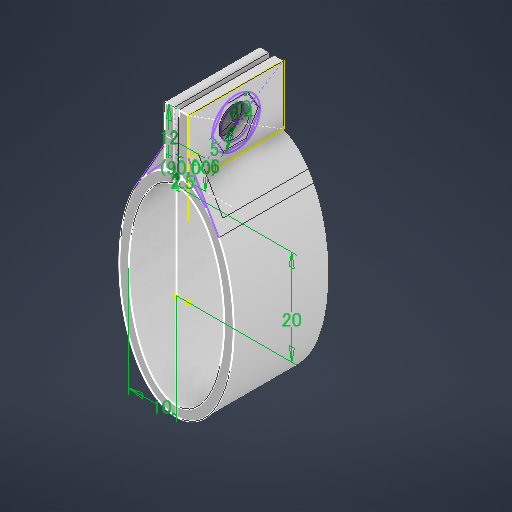
# Autodesk Inventor part: default
Saved by Autodesk Inventor 2025.2 (Build 292293000, 293)
## iProperties
Created: 2024-07-26
Part Number: default
Material: 一般
Document SubType Name: Modeling
Designer: ktamu
Density: 1 g/cm^3
Appearance: 既定
Author: ktamu
Autodesk Inventor part; units mm, degrees
note: some values were not read from the file. Chosen so that the rebuilt part matches the saved one: offset side.
ref_plane "YZ Plane" through (0, 0, 0) normal (1, 0, 0) x (0, 1, 0)
ref_plane "XZ Plane" through (0, 0, 0) normal (0, 1, 0) x (-1, 0, 0)
ref_plane "XY Plane" through (0, 0, 0) normal (0, 0, 1) x (1, 0, 0)
sketch "スケッチ1" plane through (0, 0, 0) normal (0, 0, 1) x (1, 0, 0)
  ellipse E0 centre (0, 0) end of major axis (0, -20) minor radius 10
  line L0 (0, 0) -> (0, 22)
  line L1 (0, 0) -> (0, -22)
  line L2 (0, 22) -> (0, 34)
  line L3 (0, 22) -> (12, 22) construction
  line L4 (0, 34) -> (2.5, 34)
  line L5 (2.5, 34) -> (2.5, 22)
  line L6 (2.5, 22) -> (0, 22)
  line L7 (0, 22) -> (0, 34)
  line L8 (0, 34) -> (-2.5, 34)
  line L9 (-2.5, 34) -> (-2.5, 22)
  line L10 (-2.5, 22) -> (0, 22)
  line L11 (-0.5, 34) -> (0.5, 34)
  line L12 (0.5, 34) -> (0.5, 22)
  line L13 (0.5, 22) -> (-0.5, 22)
  line L14 (-0.5, 22) -> (-0.5, 34)
  line L15 (-0.5, 34) -> (0.5, 22) construction
  line L16 (0.5, 34) -> (-0.5, 22) construction
  line L17 (2.5, 26.1957) -> (8.883, 14.9903)
  line L18 (-2.5, 26.1957) -> (-8.883, 14.9903)
  line L19 (-0.5, 22) -> (-0.5, 19.975)
  line L20 (0.5, 22) -> (0.5, 19.975)
  line L21 (-6.1194, 19.0632) -> (-2.5, 23.108)
  line L22 (6.1194, 19.0632) -> (2.5, 23.108)
  line L23 (-2.5, 22) -> (-2.5, 21.4925)
  line L24 (2.5, 22) -> (2.5, 21.3781)
  spline S0 degree 5 poles (0, -22) (1.1169, -22.0001) (2.2373, -21.7769) (3.2884, -21.3301) (5.3155, -20.0562) (6.9198, -18.2708) (7.6546, -17.2439) (9.0536, -14.8879) (10.0679, -12.3406) (10.5239, -10.9338) (11.3093, -7.9323) (11.7649, -4.8627) (11.9216, -3.2452) (12.0784, 0) (11.9216, 3.2451) (11.765, 4.8626) (11.3092, 7.9322) (10.524, 10.9338) (10.0678, 12.3407) (9.0538, 14.888) (7.6543, 17.244) (6.9201, 18.2709) (5.3148, 20.0562) (3.2891, 21.3301) (2.2357, 21.777) (0, 22.223) (-2.2357, 21.777) (-3.2891, 21.3301) (-5.3148, 20.0562) (-6.9201, 18.2709) (-7.6543, 17.244) (-9.0538, 14.888) (-10.0678, 12.3407) (-10.524, 10.9338) (-11.3092, 7.9322) (-11.765, 4.8626) (-11.9216, 3.2451) (-12.0784, 0) (-11.9216, -3.2452) (-11.7649, -4.8627) (-11.3093, -7.9323) (-10.5239, -10.9338) (-10.0679, -12.3406) (-9.0536, -14.8879) (-7.6546, -17.2439) (-6.9198, -18.2708) (-5.3155, -20.0562) (-3.2884, -21.3301) (-2.2373, -21.7769) (-1.1169, -22.0001) (0, -22) knots 0 0 0 0 0 0 0.051048 0.051048 0.051048 0.108461 0.108461 0.108461 0.175874 0.175874 0.175874 0.25 0.25 0.25 0.324124 0.324124 0.324124 0.391541 0.391541 0.391541 0.448952 0.448952 0.448952 0.5 0.5 0.5 0.551048 0.551048 0.551048 0.608459 0.608459 0.608459 0.675876 0.675876 0.675876 0.75 0.75 0.75 0.824126 0.824126 0.824126 0.891539 0.891539 0.891539 0.948952 0.948952 0.948952 1 1 1 1 1 1
  point P0 (0, 28)
  point P1 (1.25, 22)
  point P2 (-7.7502, 16.9789)
  point P3 (-8.883, 14.9903)
  point P4 (7.7502, 16.9789)
  point P5 (-0.5, 21.9822)
  point P6 (0.5, 21.9822)
  point P7 (-2.5, 21.5469)
  point P8 (2.5, 21.5469)
  dimension "d0" = 10
  dimension "d1" = 20
  dimension "d2" = 2
  dimension "d3" = 12
  dimension "d4" = 90
  dimension "d5" = 2.5
  dimension "d6" = 6
  dimension "d7" = 1
  constraints: 50 end point, 6 symmetric about line, 5 point on line, 4 horizontal, 4 midpoint, 4 parallel, 4 vertical, 3 perpendicular, 2 collinear, 1 coincident, 9 other
  measures "d3" distance of L0.end L2.end
  measures "d4" angle of L3 L2
  measures "d5" distance of L5.end L6.end
  measures "d6" vertical distance of point (1.25, 22) point (0, 28)
  measures "d7" distance of L12.end L13.end
extrude "押し出し1" add sketch "スケッチ1" against normal blind 20 contours L1 S0 L18 L19 E0 | E0 L20 S0 L17 L1 | E0 L0 S0 L20 | L19 S0 L0 E0 | L12 L4 L5 L6 | L10 L9 L8 L14
extrude "押し出し2" add sketch "スケッチ1" against normal blind 2 contours S0 L6 L20 | L20 L6 L24 S0 | S0 L23 L10 L19 | L19 L10 S0 | L24 L5 L22 S0 | S0 L21 L9 L23 | S0 L22 L5 L17 | L18 L9 L21 S0
extrude "押し出し3" cut sketch "スケッチ1" against normal through all contours E0 L0 S0 L20 | L19 S0 L0 E0
fillet "フィレット1" radius 1.3 2 edges at (0.5, 19.975, -10) (-0.5, 19.975, -10)
extrude "押し出し4" add sketch "スケッチ1" against normal blind 20 contours L20 L6 L24 S0 | S0 L23 L10 L19
sketch "スケッチ2" plane through (2.5, 26.1957, 0) normal (1, 0, 0) x (0, 0, -1)
  line L0 (2, -4.6488) -> (2, 0) projected
  line L1 (20, 7.8043) -> (20, -4.6488) projected
  line L2 (0, 7.8043) -> (20, 7.8043) projected
  line L3 (0, 0) -> (0, 7.8043) projected
  line L4 (0, 0) -> (2, 0) projected
  line L5 (0, 7.8043) -> (20, -4.6488) construction
  line L6 (20, 7.8043) -> (0, -4.6488) construction
  line L7 (0, 0) -> (0, -11.2054) projected
  circle A0 centre (10, 1.5777) radius 3.2
  circle A1 centre (10, 1.5777) radius 5
  line L8 (14.2445, 4.2206) -> (10, 1.5777)
  line L9 (5, 1.5777) -> (7.5, -2.7524)
  line L10 (7.5, -2.7524) -> (12.5, -2.7524)
  line L11 (12.5, -2.7524) -> (15, 1.5777)
  line L12 (15, 1.5777) -> (12.5, 5.9079)
  line L13 (12.5, 5.9079) -> (7.5, 5.9079)
  line L14 (7.5, 5.9079) -> (5, 1.5777)
  point P0 (0, -26.1957)
  dimension "d18" = 10
  dimension "d17" = 6.4
  dimension "d19" = 5
  constraints: 18 end point, 3 midpoint, 2 parallel, 1 centre point, 1 coincident, 1 collinear, 1 horizontal, 1 horizontal alignment, 1 point on line, 9 other
  measures "d17" diameter of A0
  measures "d19" distance of L9.start L9.end
extrude "押し出し5" cut sketch "スケッチ2" against normal through all contours A0
extrude "押し出し6" cut sketch "スケッチ2" against normal blind 0.4 contours L11 L10 L9 L14 L13 L12
equation "\"d6\" = 0.5 * d3"
